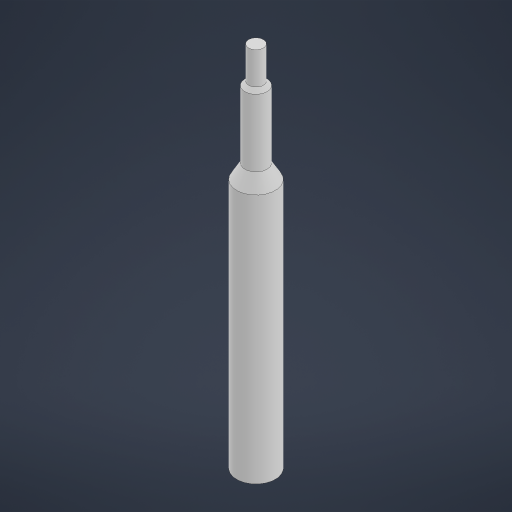
# Autodesk Inventor part: R217.13-023050CC06K 1630
Saved by Autodesk Inventor 2024.1 (Build 281209000, 209)
## iProperties
Created: 2023-11-19
Part Number: R217.13-023050CC06K 1630
Material: Generic
Document SubType Name: Modeling
Designer: fablabadmin
Density: 1 g/cm^3
Appearance: Default
Author: fablabadmin
Autodesk Inventor part; units mm, degrees
ref_plane "YZ Plane" through (0, 0, 0) normal (1, 0, 0) x (0, 1, 0)
ref_plane "XZ Plane" through (0, 0, 0) normal (0, 1, 0) x (-1, 0, 0)
ref_plane "XY Plane" through (0, 0, 0) normal (0, 0, 1) x (1, 0, 0)
sketch "Sketch1" plane through (0, 0, 0) normal (0, 0, 1) x (1, 0, 0)
  line L0 (-3.6, 0) -> (0.6, 0) construction
  line L1 (0, 0) -> (-3, 0)
  line L2 (-3, 0) -> (-3, 38.8)
  line L3 (-3, 38.8) -> (-1.725, 41.0084)
  line L4 (-1.725, 41.0084) -> (-1.725, 51.425)
  line L5 (-1.725, 51.425) -> (-1.15, 52)
  line L6 (-1.15, 52) -> (-1.15, 57)
  line L7 (-1.15, 57) -> (0, 57)
  line L8 (0, 57) -> (0, 0)
  dimension "d0" = 57
  dimension "d10" = 5
  dimension "d13" = 5.575
  dimension "d16" = 38.8
  dimension "d17" = 6
  dimension "d18" = 3.45
  dimension "d19" = 2.3
  dimension "d20" = 30
  dimension "d21" = 45
  constraints: 16 end point, 2 parallel, 1 perpendicular, 1 point on line, 1 vertical
  measures "d0" vertical distance of L1.end L6.end
  measures "d10" distance of L5.end L6.end
  measures "d13" vertical distance of L4.end L6.end
  measures "d16" distance of L1.end L2.end
  measures "d17" diameter of L2 L8
  measures "d18" diameter of L4 L8
  measures "d19" diameter of L6 L8
  measures "d20" angle of L8 L3
  measures "d21" angle of L8 L5
revolve "Revolution1" add sketch "Sketch1" angle 360 about axis through (0, 57, 0) along (0, -1, 0)
body "Solid1"
